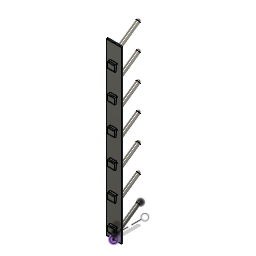
spool_holder_7_row (Autodesk Fusion 360 design; units mm, degrees)
Autodesk Fusion 360 part; units mm, degrees
sketch "Sketch1" plane through (0, 0, 0) normal (0, 0, 1) x (1, 0, 0)
  line L0 (0, 0) -> (20, 0)
  line L1 (20, 0) -> (20, 226.2)
  line L2 (20, 226.2) -> (0, 226.2)
  line L3 (0, 226.2) -> (0, 0)
  line L4 (10, 0) -> (10, 226.2)
  line L5 (5.5, 16.35) -> (14.5, 16.35)
  line L6 (14.5, 16.35) -> (14.5, 14.35)
  line L7 (14.5, 14.35) -> (5.5, 14.35)
  line L8 (5.5, 14.35) -> (5.5, 16.35)
  line L9 (5.5, 14.35) -> (14.5, 14.35)
  line L10 (14.5, 14.35) -> (14.5, 7.35)
  line L11 (14.5, 7.35) -> (5.5, 7.35)
  line L12 (5.5, 7.35) -> (5.5, 14.35)
  line L13 (14.5, 45.05) -> (5.5, 45.05)
  line L14 (14.5, 54.05) -> (14.5, 52.05)
  line L15 (14.5, 52.05) -> (5.5, 52.05)
  line L16 (5.5, 54.05) -> (14.5, 54.05)
  line L17 (5.5, 52.05) -> (14.5, 52.05)
  line L18 (14.5, 52.05) -> (14.5, 45.05)
  line L19 (5.5, 52.05) -> (5.5, 54.05)
  line L20 (5.5, 45.05) -> (5.5, 52.05)
  line L21 (14.5, 82.75) -> (5.5, 82.75)
  line L22 (14.5, 91.75) -> (14.5, 89.75)
  line L23 (14.5, 89.75) -> (5.5, 89.75)
  line L24 (5.5, 91.75) -> (14.5, 91.75)
  line L25 (5.5, 89.75) -> (14.5, 89.75)
  line L26 (14.5, 89.75) -> (14.5, 82.75)
  line L27 (5.5, 89.75) -> (5.5, 91.75)
  line L28 (5.5, 82.75) -> (5.5, 89.75)
  line L29 (14.5, 120.45) -> (5.5, 120.45)
  line L30 (14.5, 129.45) -> (14.5, 127.45)
  line L31 (14.5, 127.45) -> (5.5, 127.45)
  line L32 (5.5, 129.45) -> (14.5, 129.45)
  line L33 (5.5, 127.45) -> (14.5, 127.45)
  line L34 (14.5, 127.45) -> (14.5, 120.45)
  line L35 (5.5, 127.45) -> (5.5, 129.45)
  line L36 (5.5, 120.45) -> (5.5, 127.45)
  line L37 (14.5, 158.15) -> (5.5, 158.15)
  line L38 (14.5, 167.15) -> (14.5, 165.15)
  line L39 (14.5, 165.15) -> (5.5, 165.15)
  line L40 (5.5, 167.15) -> (14.5, 167.15)
  line L41 (5.5, 165.15) -> (14.5, 165.15)
  line L42 (14.5, 165.15) -> (14.5, 158.15)
  line L43 (5.5, 165.15) -> (5.5, 167.15)
  line L44 (5.5, 158.15) -> (5.5, 165.15)
  line L45 (14.5, 195.85) -> (5.5, 195.85)
  line L46 (14.5, 204.85) -> (14.5, 202.85)
  line L47 (14.5, 202.85) -> (5.5, 202.85)
  line L48 (5.5, 204.85) -> (14.5, 204.85)
  line L49 (5.5, 202.85) -> (14.5, 202.85)
  line L50 (14.5, 202.85) -> (14.5, 195.85)
  line L51 (5.5, 202.85) -> (5.5, 204.85)
  line L52 (5.5, 195.85) -> (5.5, 202.85)
  dimension "d4" = 226.2
  dimension "d5" = 20
  dimension "d6" = 9
  dimension "d7" = 2
  dimension "d8" = 9
  dimension "d9" = 14.35
  dimension "d10" = 7
  dimension "d11" = 9
  dimension "d14" = 28.7
  dimension "d15" = 37.7
  constraint horizontal L0
  constraint vertical L1
  constraint horizontal L2
  constraint vertical L3
  constraint coincident L0.start L3.end
  constraint midpoint L0 L4.start
  constraint midpoint L2 L4.end
  constraint horizontal L5
  constraint vertical L6
  constraint horizontal L7
  constraint vertical L8
  constraint horizontal L9
  constraint vertical L10
  constraint horizontal L11
  constraint vertical L12
  measures "d4" distance of L0.start L2.end
  measures "d5" distance of L0.start L0.end
  measures "d6" distance of L5.start L5.end
  measures "d7" distance of L5.start L7.end
  measures "d9" distance of L0 L7
  measures "d10" distance of L7.end L11.end
  measures "d11" distance of L10.end L11.end
extrude "Extrude1" add sketch "Sketch1" against normal blind 2
extrude "Extrude2" add sketch "Sketch1" along normal blind 3.5 contours L4 L5 L7 L8 L9 | L4 L5 L6 L7 L9 | L4 L46 L47 L48 L49 | L4 L47 L48 L49 L51 | L4 L15 L16 L17 L19 | L4 L14 L15 L16 L17 | L4 L38 L39 L40 L41 | L4 L39 L40 L41 L43 | L4 L23 L24 L25 L27 | L4 L22 L23 L24 L25 | L4 L30 L31 L32 L33 | L4 L31 L32 L33 L35
extrude "Extrude3" add sketch "Sketch1" against normal blind 2 from surface at 3.5 contours L4 L7 L9 L11 L12 | L4 L7 L9 L10 L11 | L4 L45 L47 L49 L50 | L4 L45 L47 L49 L52 | L4 L13 L15 L17 L20 | L4 L13 L15 L17 L18 | L4 L37 L39 L41 L42 | L4 L37 L39 L41 L44 | L4 L21 L23 L25 L28 | L4 L21 L23 L25 L26 | L4 L29 L31 L33 L34 | L4 L29 L31 L33 L36
fillet "Fillet1" radius 1 18 edges at (10, 16.35, 3.5) (10, 7.35, 1.5) (10, 7.35, 3.5) (10, 45.05, 1.5) (10, 45.05, 3.5) (10, 54.05, 3.5) (10, 82.75, 1.5) (10, 82.75, 3.5) (10, 91.75, 3.5) (10, 120.45, 1.5) (10, 120.45, 3.5) (10, 129.45, 3.5) (10, 158.15, 1.5) (10, 158.15, 3.5) (10, 167.15, 3.5) (10, 195.85, 1.5) (10, 195.85, 3.5) (10, 204.85, 3.5)
ref_plane "WorkPlane1" through (10, 113.1, -1) normal (1, 0, 0) x (0, -1, 0)
sketch "Sketch2" plane through (10, 0, 0) normal (1, 0, 0) x (0, 0, -1)
  line L0 (2, 5) -> (3.847, 5)
  line L1 (9.5828, 6.8085) -> (35.6703, 25.0752)
  line L2 (7, 5) -> (41.421, 5) construction
  line L3 (0, 0) -> (2, 0)
  arc A0 (3.847, 5) -> (9.5828, 6.8085) centre (3.847, 15) ccw
  dimension "d26" = 5
  dimension "d27" = 35
  dimension "d28" = 35
  dimension "d29" = 5
  dimension "d30" = 2
  dimension "d40" = 10
  constraint horizontal L0
  constraint horizontal L2
  constraint coincident L2.start L0
  constraint coincident L2.start L1
  constraint tangent L0 A0
  constraint tangent L1 A0
  measures "d26" distance of L0.start L2.start
  measures "d27" distance of L2.start L1.end
  measures "d28" angle of L1 L2
  measures "d29" distance of L0 L3
  measures "d30" horizontal distance of L3.start L0.start
  measures "d40" radius of A0
sketch "Sketch3" plane through (0, 0, -2) normal (0, 0, -1) x (-1, 0, 0)
  line L0 (0, 0) -> (0, 226.2)
  line L1 (0, 226.2) -> (-20, 226.2)
  line L2 (-20, 226.2) -> (-20, 0)
  line L3 (-20, 0) -> (0, 0)
  circle A0 centre (-10, 7) radius 2.5
  dimension "d31" = 5
  dimension "d32" = 7
  dimension "d33" = 10
  measures "d31" diameter of A0
  measures "d32" distance of L3 A0.centre
  measures "d33" distance of L2 A0.centre
sweep "Sweep1" add profiles "Sketch3" path "Sketch2" along L0 A0 L1 section 1 contours A0
fillet "Fillet2" radius 2.5 1 edges at (12.3308, 25.9729, -35.0417)
fillet "Fillet3" radius 2 1 edges at (12.3308, 7.904, -2)
pattern_linear "R-Pattern1" count 7 spacing 35 along (0, 1, 0) of "Sweep1", "Fillet2", "Fillet3"
chamfer "Chamfer1" distance 0.5 distance2 6 6 edges at (10, 202.85, 1.5) (10, 165.15, 1.5) (10, 127.45, 1.5) (10, 89.75, 1.5) (10, 52.05, 1.5) (10, 14.35, 1.5) measured on face at (11.5, 202.85, 0.5) measured on face at (11.5, 165.15, 0.5) measured on face at (11.5, 127.45, 0.5) measured on face at (11.5, 89.75, 0.5) measured on face at (11.5, 52.05, 0.5) measured on face at (11.5, 14.35, 0.5)
equation "square_hole_dim = 9 mm"
equation "distance_between_holes = 28.7 mm"
equation "rod_dia = 5 mm"
equation "d4 = square_hole_dim * 6 + distance_between_holes * 6"
equation "d6 = square_hole_dim"
equation "d8 = square_hole_dim"
equation "d9 = distance_between_holes / 2"
equation "d10 = square_hole_dim - 2 mm"
equation "d11 = square_hole_dim"
equation "d14 = distance_between_holes"
equation "d15 = distance_between_holes + square_hole_dim"
equation "distance_between_rods = 35 mm"
equation "d45 = distance_between_rods"
